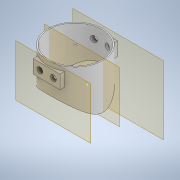
# Autodesk Inventor part: Part7
Saved by Autodesk Inventor 2020 (Build 240168000, 168)
## iProperties
Created: 2022-04-08
Part Number: Part7
Material: Generic
Document SubType Name: Modeling
Designer: Mic
Density: 1 g/cm^3
Appearance: Default
Author: Mic
Autodesk Inventor part; units mm, degrees
ref_plane "YZ Plane" through (0, 0, 0) normal (1, 0, 0) x (0, 1, 0)
ref_plane "XZ Plane" through (0, 0, 0) normal (0, 1, 0) x (-1, 0, 0)
sketch "Sketch1" plane through (0, 0, 0) normal (0, 1, 0) x (-1, 0, 0)
  circle A0 centre (20.8145, -14.703) radius 14.1152
  circle A1 centre (20.8145, -14.703) radius 13.5152
  point P0 (0, 0)
  dimension "d0" = 0.6
  constraints: 2 centre point
  measures "d0" radial gap between concentric circles of A0 A1
extrude "Extrusion1" add sketch "Sketch1" along normal blind 24
ref_plane "Work Plane1" through (0, 0, -29) normal (0, 0, 1) x (1, 0, 0)
sketch "Sketch3" plane through (0, 0, 0) normal (1, 0, 0) x (0, 1, 0)
  point P0 (0, 0)
sketch "Sketch4" plane through (0, 0, 0) normal (0, 0, 1) x (1, 0, 0)
  line L0 (-34.9297, 0) -> (-34.9297, 24) projected
  line L1 (-6.6992, 0) -> (-6.6992, 24) projected
  line L2 (-34.9297, 18.2399) -> (-20.8145, 18.2399) construction
  line L3 (-20.8145, 18.2399) -> (-6.6992, 18.2399) construction
  line L4 (-13.9813, 14.7399) -> (-27.6476, 14.7399)
  line L5 (-27.6476, 14.7399) -> (-27.6476, 21.7399)
  line L6 (-27.6476, 21.7399) -> (-13.9813, 21.7399)
  line L7 (-13.9813, 21.7399) -> (-13.9813, 14.7399)
  line L8 (-13.9813, 14.7399) -> (-27.6476, 21.7399) construction
  line L9 (-27.6476, 14.7399) -> (-13.9813, 21.7399) construction
  point P0 (0, 0)
  dimension "d14" = 7
  constraints: 16 end point, 3 point on line, 2 horizontal, 2 midpoint, 2 parallel, 1 collinear, 1 perpendicular
  measures "d14" distance of L6.end L4.start
extrude "Extrusion3" add sketch "Sketch4" against normal up to surface
sketch "Sketch5" plane through (-20.8145, 24, -14.703) normal (0, 1, 0) x (1, 0, 0)
  point P0 (20.8145, -14.703)
  point P1 (0, 0)
ref_plane "Work Plane2" through (-20.8145, 24, -14.703) normal (0, 0, 1) x (1, 0, 0)
mirror "Mirror1" about plane through (-20.8145, 24, -14.703) normal (0, 0, 1) of "Extrusion3"
sketch "Sketch6" plane through (0, 0, 0) normal (0, 0, 1) x (1, 0, 0)
  line L0 (-13.9813, 14.7399) -> (-13.9813, 21.7399) projected
  line L1 (-13.9813, 21.7399) -> (-27.6476, 21.7399) projected
  line L2 (-27.6476, 21.7399) -> (-27.6476, 14.7399) projected
  line L3 (-27.6476, 14.7399) -> (-13.9813, 14.7399) projected
  line L4 (-17.3456, 21.7399) -> (-17.3456, 18.2399) construction
  line L5 (-17.3456, 18.2399) -> (-17.3456, 14.7399) construction
  line L6 (-24.2833, 21.7399) -> (-24.2833, 18.2399) construction
  line L7 (-24.2833, 18.2399) -> (-24.2833, 14.7399) construction
  line L8 (-17.3456, 18.2399) -> (-13.9813, 18.2399) construction
  line L9 (-13.9813, 21.7399) -> (-13.9813, 14.7399) construction
  line L10 (-24.2833, 18.2399) -> (-27.6476, 18.2399) construction
  circle A0 centre (-17.3456, 18.2399) radius 1.5
  circle A1 centre (-24.2833, 18.2399) radius 1.5
  point P0 (0, 0)
  dimension "d10" = 3
  dimension "d11" = 3
  constraints: 12 end point, 6 point on line, 3 collinear, 2 centre point, 2 coincident, 2 midpoint, 2 vertical
  measures "d10" diameter of A0
  measures "d11" diameter of A1
extrude "Extrusion4" cut sketch "Sketch6" against normal blind 72.25 contours A0 | A1
sketch "Sketch7" plane through (0, 0, 0) normal (0, 0, 1) x (1, 0, 0)
  circle A0 centre (-20.8145, -7.4962) radius 16.4655
  line L0 (-34.9297, 0) -> (-34.9297, 24) projected
  line L1 (-6.6992, 0) -> (-6.6992, 24) projected
  line L2 (-34.9297, 12) -> (-20.8145, 12)
  line L3 (-20.8145, 12) -> (-6.6992, 12)
  line L4 (-20.8145, 12) -> (-20.8145, -15.8986) construction
  point P0 (0, 0)
  dimension "d15" = 32.931
  constraints: 6 end point, 2 midpoint, 1 centre point, 1 collinear, 1 horizontal, 1 point on line, 1 vertical
  measures "d15" diameter of A0
extrude "Extrusion5" cut sketch "Sketch7" against normal blind 60.25 contours A0
body "Solid1"
